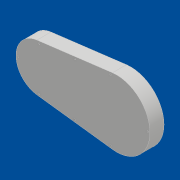
# Autodesk Inventor part: 111-base template
Saved by Autodesk Inventor 2018 (Build 220112000, 112)
## iProperties
Created: 2019-11-07
Part Number: 111-base template
Material: Generic
Document SubType Name: Modeling
Designer: Bunny320
Density: 1 g/cm^3
Appearance: Default
Author: Bunny320
Autodesk Inventor part; units mm, degrees
ref_plane "YZ Plane" through (0, 0, 0) normal (1, 0, 0) x (0, 1, 0)
ref_plane "XZ Plane" through (0, 0, 0) normal (0, 1, 0) x (-1, 0, 0)
ref_plane "XY Plane" through (0, 0, 0) normal (0, 0, 1) x (1, 0, 0)
sketch "Sketch2" plane through (0, 0, 0) normal (0, 1, 0) x (-1, 0, 0)
  circle A0 centre (0, 0) radius 40
  circle A1 centre (-141.206, 0) radius 57.5
  line L0 (4.9573, -39.6916) -> (-134.0799, -57.0567)
  line L1 (4.9573, 39.6916) -> (-134.0799, 57.0567)
  dimension "d5" = 141.206
  dimension "d6" = 80
  dimension "d7" = 115
  constraints: 4 end point, 4 point on circle, 4 tangent, 2 centre point, 1 coincident, 1 horizontal alignment
  measures "d5" distance of A1.centre point (0, 0)
  measures "d6" diameter of A0
  measures "d7" diameter of A1
extrude "Extrusion2" add sketch "Sketch2" along normal blind 4
sketch "Sketch14" plane through (0, 0, 0) normal (0, 1, 0) x (-1, 0, 0)
  arc A0 (4.9573, -39.6916) -> (4.9573, 39.6916) centre (0, 0) ccw projected
  arc A1 (5.453, -43.6608) -> (5.453, 43.6608) centre (0, 0) ccw
  arc A2 (-134.0799, 57.0567) -> (-134.0799, -57.0567) centre (-141.206, 0) ccw projected
  arc A3 (-133.5842, 61.0259) -> (-133.5842, -61.0259) centre (-141.206, 0) ccw
  line L0 (5.453, -43.6608) -> (-133.5842, -61.0259)
  line L1 (-133.5842, 61.0259) -> (5.453, 43.6608)
  line L2 (-134.0799, -57.0567) -> (4.9573, -39.6916)
  arc A4 (4.9573, -39.6916) -> (4.9573, 39.6916) centre (0, 0) ccw
  line L3 (4.9573, 39.6916) -> (-134.0799, 57.0567)
  arc A5 (-134.0799, 57.0567) -> (-134.0799, -57.0567) centre (-141.206, 0) ccw
  dimension "d53" = 4
  dimension "d54" = 4
  dimension "d55" = 4
  constraints: 8 end point, 8 point on circle, 4 centre point, 4 tangent, 2 coincident, 3 other
  measures "d53" radial gap between concentric circles of A0 A1
  measures "d54" radial gap between concentric circles of A2 A3
  measures "d55" distance between parallel lines of L2 L0
extrude "Extrusion11" add sketch "Sketch14" along normal blind 26
sketch "Sketch27" plane through (0, 4, 0) normal (0, 1, 0) x (1, 0, 0)
  line L0 (-40, 4) -> (-36, 4)
  line L1 (-36, 4) -> (-36, -4)
  line L2 (-36, -4) -> (-40, -4)
  line L3 (-40, -4) -> (-40, 4)
  line L4 (-40, 4) -> (-36, -4) construction
  line L5 (-36, 4) -> (-40, -4) construction
  arc A0 (-4.9573, 39.6916) -> (-4.9573, -39.6916) centre (0, 0) ccw projected
  line L6 (-4.9573, 39.6916) -> (134.0799, 57.0567) projected
  arc A1 (134.0799, -57.0567) -> (134.0799, 57.0567) centre (141.206, 0) ccw projected
  line L7 (194.706, 4) -> (198.706, 4)
  line L8 (198.706, 4) -> (198.706, -4)
  line L9 (198.706, -4) -> (194.706, -4)
  line L10 (194.706, -4) -> (194.706, 4)
  line L11 (194.706, 4) -> (198.706, -4) construction
  line L12 (198.706, 4) -> (194.706, -4) construction
  line L13 (134.0799, 57.0567) -> (-4.9573, 39.6916) projected
  line L14 (-4.9573, 39.6916) -> (2.981, 40.6831)
  line L15 (2.981, 40.6831) -> (3.4806, 36.6831)
  line L16 (3.4806, 36.6831) -> (-4.4577, 35.6916)
  line L17 (-4.4577, 35.6916) -> (-4.9573, 39.6916)
  line L18 (134.0799, -57.0567) -> (-4.9573, -39.6916) projected
  line L19 (-4.9573, -39.6916) -> (2.981, -40.6831)
  line L20 (2.981, -40.6831) -> (3.4768, -36.7139)
  line L21 (3.4768, -36.7139) -> (-4.4616, -35.7225)
  line L22 (-4.4616, -35.7225) -> (-4.9573, -39.6916)
  arc A2 (134.0799, -57.0567) -> (134.0799, 57.0567) centre (141.206, 0) ccw projected
  line L23 (134.0799, 57.0567) -> (126.1416, 56.0653)
  line L24 (126.1416, 56.0653) -> (126.6373, 52.0961)
  line L25 (126.6373, 52.0961) -> (134.5756, 53.0876)
  line L26 (134.5756, 53.0876) -> (134.0799, 57.0567)
  line L27 (134.0799, -57.0567) -> (126.1416, -56.0653)
  line L28 (126.1416, -56.0653) -> (126.6373, -52.0961)
  line L29 (126.6373, -52.0961) -> (134.5756, -53.0876)
  line L30 (134.5756, -53.0876) -> (134.0799, -57.0567)
  line L31 (60.5921, 47.8784) -> (68.5305, 48.8699)
  line L32 (68.5305, 48.8699) -> (69.0262, 44.9007)
  line L33 (69.0262, 44.9007) -> (61.0879, 43.9093)
  line L34 (61.0879, 43.9093) -> (60.5921, 47.8784)
  line L35 (-4.9573, -39.6916) -> (134.0799, -57.0567) projected
  line L36 (60.5921, -47.8784) -> (68.5305, -48.8699)
  line L37 (68.5305, -48.8699) -> (69.0262, -44.9007)
  line L38 (69.0262, -44.9007) -> (61.0879, -43.9093)
  line L39 (61.0879, -43.9093) -> (60.5921, -47.8784)
  point P0 (-38, 0)
  point P1 (-38, 0)
  point P2 (-38, 0)
  point P3 (196.706, 0)
  point P4 (196.706, 0)
  dimension "d147" = 8
  dimension "d148" = 4
  dimension "d152" = 4
  dimension "d153" = 8
  dimension "d155" = 8
  dimension "d156" = 4
  dimension "d157" = 8
  dimension "d159" = 4
  dimension "d160" = 8
  dimension "d161" = 4
  dimension "d162" = 8
  dimension "d163" = 4
  dimension "d181" = 8
  dimension "d182" = 4
  dimension "d183" = 8
  dimension "d184" = 4
  dimension "d188" = 58.0587
  dimension "d189" = 58.0587
  constraints: 72 end point, 16 parallel, 8 perpendicular, 8 point on line, 6 midpoint, 6 tangent, 2 horizontal, 2 horizontal alignment, 1 coincident, 1 vertical alignment
  measures "d147" distance of L0.end L1.end
  measures "d148" distance of L1.end L2.end
  measures "d152" distance of L7.start L7.end
  measures "d153" distance of L9.end L7.start
  measures "d155" distance of L15.end L16.end
  measures "d156" vertical distance of L14.end L15.end
  measures "d157" distance of L20.end L21.end
  measures "d159" distance of L19.end L20.end
  measures "d160" distance of L24.end L25.end
  measures "d161" distance of L23.end L24.end
  measures "d162" distance of L28.end L29.end
  measures "d163" distance of L27.end L28.end
  measures "d181" distance of L32.end L33.end
  measures "d182" distance of L33.end L31.start
  measures "d183" distance of L37.end L38.end
  measures "d184" distance of L38.end L36.start
  measures "d188" distance between parallel lines of L15 L34
  measures "d189" distance between parallel lines of L24 L32
extrude "Extrusion19" add sketch "Sketch27" along normal up to surface (22 mm away) contours L0 A0 L3 | L0 L1 L2 A0 | A0 L2 L3 | L6 L15 L16 L17 | L22 L21 L20 L18 | L6 L32 L33 L34 | L39 L38 L37 L18 | L6 L26 L25 L24 | L28 L29 L30 L18 | L7 L8 A1 | A1 L9 L10 L7 | L8 L9 A1
fillet "Fillet4" radius 2 32 edges at (-39.7995, 15, -4) (-36, 15, -4) (-36, 15, 4) (-39.7995, 15, 4) (-4.9573, 15, -39.6916) (-4.4577, 15, -35.6916) (3.4806, 15, -36.6831) (2.981, 15, -40.6831) (-4.9573, 15, 39.6916) (-4.4616, 15, 35.7225) (3.4768, 15, 36.7139) (2.981, 15, 40.6831) (126.6373, 15, -52.0961) (126.1416, 15, -56.0653) (134.0799, 15, -57.0567) (134.5756, 15, -53.0876) (126.1416, 15, 56.0653) (126.6373, 15, 52.0961) (134.5756, 15, 53.0876) (134.0799, 15, 57.0567) (198.5667, 15, -4) (194.706, 15, -4) (194.706, 15, 4) (198.5667, 15, 4) (61.0879, 15, -43.9093) (60.5921, 15, -47.8784) (69.0262, 15, -44.9007) (68.5305, 15, -48.8699) (60.5921, 15, 47.8784) (61.0879, 15, 43.9093) (69.0262, 15, 44.9007) (68.5305, 15, 48.8699)
sketch "Sketch28" plane through (0, 26, 0) normal (0, 1, 0) x (1, 0, 0)
  arc A0 (-4.9573, 39.6916) -> (-39.7995, 4) centre (0, 0) ccw projected
  line L0 (2.981, 40.6831) -> (126.1416, 56.0653) projected
  arc A1 (198.5667, 4) -> (134.0799, 57.0567) centre (141.206, 0) ccw projected
  line L1 (126.1416, -56.0653) -> (2.981, -40.6831) projected
  line L2 (3.4806, 36.6831) -> (2.981, 40.6831) projected
  line L3 (126.1416, 56.0653) -> (126.6373, 52.0961) projected
  line L4 (2.981, -40.6831) -> (3.4768, -36.7139) projected
  line L5 (126.6373, -52.0961) -> (126.1416, -56.0653) projected
  arc A2 (70.515, 49.1178) -> (68.7783, 46.8853) centre (70.7629, 47.1332) ccw projected
  line L6 (64.5613, 48.3742) -> (70.515, 49.1178)
  arc A3 (68.7783, -46.8853) -> (70.515, -49.1178) centre (70.7629, -47.1332) ccw projected
  line L7 (64.5613, -48.3742) -> (70.515, -49.1178)
  point P0 (-40, 0)
  point P1 (-0.9881, 40.1874)
  point P2 (130.1107, 56.561)
  point P3 (198.706, 0)
  point P4 (130.1107, -56.561)
  point P5 (-0.9881, -40.1874)
  dimension "d176" = 4
  dimension "d177" = 4
  dimension "d178" = 4
  dimension "d179" = 4
  dimension "d186" = 6
  dimension "d187" = 6
  constraints: 4 end point, 4 point on line, 2 collinear, 2 horizontal alignment, 2 midpoint, 2 point on circle, 2 tangent
  measures "d176" distance from line of L3 point (130.111, 56.561)
  measures "d177" distance from line of L5 point (130.111, -56.561)
  measures "d178" distance from line of L4 point (-0.988, -40.187)
  measures "d179" distance from line of point (-0.988, 40.187) L2
  measures "d186" distance of L7.start L7.end
  measures "d187" distance of L6.start L6.end
hole "Hole7" at (-40, 26, 0) at (-0.9881, 26, -40.1874) at (130.1107, 26, -56.561) at (198.706, 26, 0) at (130.1107, 26, 56.561) at (-0.9881, 26, 40.1874) at (64.5613, 26, -48.3742) at (64.5613, 26, 48.3742) direction (0, -1, 0) diameter 2.459 end through all thread size "M3x0.5" class "6H" standard "ISO Metric profile"
equation "\"d53\" = d54"
equation "\"d55\" = d54"
equation "\"d155\" = d147"
equation "\"d156\" = d148"
equation "\"d157\" = d147"
equation "\"d159\" = d148"
equation "\"d160\" = d147"
equation "\"d161\" = d148"
equation "\"d162\" = d147"
equation "\"d163\" = d148"
body "Solid2"
